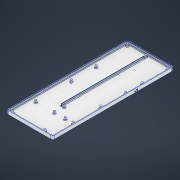
# Autodesk Inventor part: Base
Saved by Autodesk Inventor 2022 (Build 260153000, 153)
## iProperties
Created: 2021-09-21
Part Number: Base
Material: アルミニウム 6061
Document SubType Name: Modeling
Designer: shiok
Density: 2.7 g/cm^3
Appearance: アルミニウム - フラット
Author: shiok
Autodesk Inventor part; units mm, degrees
ref_plane "YZ Plane" through (0, 0, 0) normal (1, 0, 0) x (0, 1, 0)
ref_plane "XZ Plane" through (0, 0, 0) normal (0, 1, 0) x (-1, 0, 0)
ref_plane "XY Plane" through (0, 0, 0) normal (0, 0, 1) x (1, 0, 0)
ref_plane "作業平面5" through (0, 0, 0) normal (0, -1, 0) x (1, 0, 0)
sketch "スケッチ16" plane through (0, 0, 0) normal (0, -1, 0) x (1, 0, 0)
  line L0 (-65.58, -185.7375) -> (65.58, -185.7375)
  line L1 (71.12, -180.1975) -> (71.12, 180.1975)
  line L2 (65.58, 185.7375) -> (-65.58, 185.7375)
  line L3 (-71.12, 180.1975) -> (-71.12, -180.1975)
  arc A0 (-71.12, -180.1975) -> (-65.58, -185.7375) centre (-65.58, -180.1975) ccw
  arc A1 (65.58, -185.7375) -> (71.12, -180.1975) centre (65.58, -180.1975) ccw
  arc A2 (71.12, 180.1975) -> (65.58, 185.7375) centre (65.58, 180.1975) ccw
  arc A3 (-65.58, 185.7375) -> (-71.12, 180.1975) centre (-65.58, 180.1975) ccw
  line L4 (-65.58, -180.1975) -> (65.58, 180.1975)
  line L5 (-65.58, 180.1975) -> (65.58, -180.1975)
  point P0 (0, 0)
  point P1 (71.12, 185.7375)
  point P2 (71.12, -185.7375)
  point P3 (-71.12, 185.7375)
  point P4 (0, 0)
  point P5 (0, 0)
  dimension "d108" = 142.24
  dimension "d109" = 371.475
  dimension "d110" = 5.54
  constraints: 12 end point, 8 point on circle, 8 tangent, 6 point on line, 4 centre point, 3 equal radius, 3 midpoint, 2 parallel, 1 coincident, 1 horizontal, 1 perpendicular
  measures "d108" distance of point (-71.12, 185.738) point (71.12, 185.738)
  measures "d109" distance of point (71.12, 185.738) point (71.12, -185.738)
  measures "d110" radius of A0
extrude "押し出し12" add sketch "スケッチ16" against normal blind 2.54
sketch "スケッチ17" plane through (0, 2.54, 0) normal (0, 1, 0) x (1, 0, 0)
  line L0 (65.58, 183.1975) -> (-65.58, 183.1975)
  line L1 (-68.58, 180.1975) -> (-68.58, -180.1975)
  line L2 (-65.58, -183.1975) -> (65.58, -183.1975)
  line L3 (68.58, -180.1975) -> (68.58, 180.1975)
  arc A0 (68.58, 180.1975) -> (65.58, 183.1975) centre (65.58, 180.1975) ccw
  arc A1 (65.58, -183.1975) -> (68.58, -180.1975) centre (65.58, -180.1975) ccw
  arc A2 (-68.58, -180.1975) -> (-65.58, -183.1975) centre (-65.58, -180.1975) ccw
  arc A3 (-65.58, 183.1975) -> (-68.58, 180.1975) centre (-65.58, 180.1975) ccw
  line L4 (71.12, 180.1975) -> (71.12, -180.1975)
  arc A4 (65.58, -185.7375) -> (71.12, -180.1975) centre (65.58, -180.1975) ccw
  line L5 (65.58, -185.7375) -> (-65.58, -185.7375)
  arc A5 (-71.12, -180.1975) -> (-65.58, -185.7375) centre (-65.58, -180.1975) ccw
  line L6 (-71.12, -180.1975) -> (-71.12, 180.1975)
  arc A6 (-65.58, 185.7375) -> (-71.12, 180.1975) centre (-65.58, 180.1975) ccw
  line L7 (-65.58, 185.7375) -> (65.58, 185.7375)
  arc A7 (71.12, 180.1975) -> (65.58, 185.7375) centre (65.58, 180.1975) ccw
  line L8 (-65.58, 180.1975) -> (65.58, -180.1975) construction
  line L9 (-65.58, -180.1975) -> (65.58, 180.1975) construction
  circle A8 centre (62.23, 176.8475) radius 3
  circle A9 centre (63.5, 96.8375) radius 3
  circle A10 centre (63.5, 46.0375) radius 3
  circle A11 centre (62.23, -28.8925) radius 3
  circle A12 centre (62.23, -113.9825) radius 3
  circle A13 centre (38.1, -113.9825) radius 3
  circle A14 centre (38.1, -176.8475) radius 3
  circle A15 centre (-62.23, -176.8475) radius 3
  circle A16 centre (4.445, -113.9825) radius 3
  circle A17 centre (4.445, -83.5025) radius 3
  circle A18 centre (-52.705, -113.9825) radius 3
  circle A19 centre (-52.705, -4.7625) radius 3
  circle A20 centre (-52.705, 71.4375) radius 3
  circle A21 centre (-62.23, 176.8475) radius 3
  circle A22 centre (-5.08, 176.8475) radius 3
  point P0 (0, 0)
  point P1 (0, 0)
  point P2 (0, 0)
  point P3 (0, 0)
  point P4 (52.07, 166.6875)
  dimension "d113" = 3
  dimension "d114" = 2.54
  dimension "d115" = 366.395
  dimension "d116" = 137.16
  dimension "d117" = 16.51
  dimension "d118" = 16.51
  dimension "d119" = 10.16
  dimension "d120" = 10.16
  dimension "d121" = 1.27
  dimension "d122" = 1.27
  dimension "d123" = 80.01
  dimension "d124" = 50.8
  dimension "d125" = 74.93
  dimension "d126" = 85.09
  dimension "d127" = 6
  dimension "d128" = 6
  dimension "d129" = 6
  dimension "d130" = 6
  dimension "d131" = 6
  dimension "d132" = 24.13
  dimension "d133" = 62.865
  dimension "d134" = 100.33
  dimension "d135" = 62.865
  dimension "d136" = 9.525
  dimension "d137" = 6
  dimension "d138" = 6
  dimension "d139" = 57.15
  dimension "d140" = 76.2
  dimension "d141" = 6
  dimension "d142" = 6
  dimension "d143" = 109.22
  dimension "d144" = 6
  dimension "d145" = 6
  dimension "d146" = 6
  dimension "d147" = 6
  dimension "d148" = 6
  dimension "d149" = 6
  dimension "d150" = 30.48
  dimension "d151" = 33.655
  constraints: 23 centre point, 20 end point, 16 point on circle, 8 tangent, 7 vertical alignment, 5 horizontal alignment, 4 parallel, 3 equal radius, 3 midpoint, 2 perpendicular, 1 coincident, 1 horizontal, 7 other
  measures "d113" radius of A0
  measures "d114" distance between parallel lines of L3 L4
  measures "d115" distance between parallel lines of L2 L0
  measures "d116" distance between parallel lines of L1 L3
  measures "d117" distance from line of point (52.07, 166.688) L3
  measures "d118" distance from line of L0 point (52.07, 166.688)
  measures "d119" horizontal distance of A8.centre point (52.07, 166.688)
  measures "d120" horizontal distance of point (52.07, 166.688) A8.centre
  measures "d121" horizontal distance of A9.centre A8.centre
  measures "d122" horizontal distance of A11.centre A10.centre
  measures "d123" vertical distance of A9.centre A8.centre
  measures "d124" distance of A9.centre A10.centre
  measures "d125" vertical distance of A10.centre A11.centre
  measures "d126" distance of A12.centre A11.centre
  measures "d127" diameter of A8
  measures "d128" diameter of A9
  measures "d129" diameter of A10
  measures "d130" diameter of A11
  measures "d131" diameter of A12
  measures "d132" distance of A13.centre A12.centre
  measures "d133" distance of A14.centre A13.centre
  measures "d134" distance of A15.centre A14.centre
  measures "d135" vertical distance of A18.centre A15.centre
  measures "d136" horizontal distance of A18.centre A15.centre
  measures "d137" diameter of A21
  measures "d138" diameter of A22
  measures "d139" distance of A21.centre A22.centre
  measures "d140" distance of A19.centre A20.centre
  measures "d141" diameter of A20
  measures "d142" diameter of A19
  measures "d143" distance of A18.centre A19.centre
  measures "d144" diameter of A13
  measures "d145" diameter of A14
  measures "d146" diameter of A15
  measures "d147" diameter of A18
  measures "d148" diameter of A17
  measures "d149" diameter of A16
  measures "d150" distance of A17.centre A16.centre
  measures "d151" distance of A13.centre A16.centre
extrude "押し出し13" add sketch "スケッチ17" along normal blind 6.4 contours A8 | A9 | A10 | A11 | A12 | A13 | A14 | A15 | A16 | A17 | A18 | A19 | A20 | A21 | A22
sketch "スケッチ18" plane through (0, 2.54, 0) normal (0, 1, 0) x (1, 0, 0)
  line L0 (-65.58, -185.7375) -> (65.58, -185.7375)
  line L1 (71.12, -180.1975) -> (71.12, 180.1975)
  line L2 (65.58, 185.7375) -> (-65.58, 185.7375)
  line L3 (-71.12, 180.1975) -> (-71.12, -180.1975)
  arc A0 (-71.12, -180.1975) -> (-65.58, -185.7375) centre (-65.58, -180.1975) ccw
  arc A1 (65.58, -185.7375) -> (71.12, -180.1975) centre (65.58, -180.1975) ccw
  arc A2 (71.12, 180.1975) -> (65.58, 185.7375) centre (65.58, 180.1975) ccw
  arc A3 (-65.58, 185.7375) -> (-71.12, 180.1975) centre (-65.58, 180.1975) ccw
  line L4 (-65.58, -180.1975) -> (65.58, 180.1975)
  line L5 (-65.58, 180.1975) -> (65.58, -180.1975)
  line L6 (68.58, 180.1975) -> (68.58, -180.1975)
  arc A4 (65.58, -183.1975) -> (68.58, -180.1975) centre (65.58, -180.1975) ccw
  line L7 (65.58, -183.1975) -> (-65.58, -183.1975)
  arc A5 (-68.58, -180.1975) -> (-65.58, -183.1975) centre (-65.58, -180.1975) ccw
  line L8 (-68.58, -180.1975) -> (-68.58, 180.1975)
  arc A6 (-65.58, 183.1975) -> (-68.58, 180.1975) centre (-65.58, 180.1975) ccw
  line L9 (-65.58, 183.1975) -> (65.58, 183.1975)
  arc A7 (68.58, 180.1975) -> (65.58, 183.1975) centre (65.58, 180.1975) ccw
  point P0 (0, 0)
  point P1 (0, 0)
  point P2 (71.12, 185.7375)
  point P3 (71.12, -185.7375)
  point P4 (-71.12, 185.7375)
  point P5 (0, 0)
  point P6 (0, 0)
  dimension "d154" = 142.24
  dimension "d155" = 371.475
  dimension "d156" = 5.54
  dimension "d157" = 2.54
  constraints: 20 end point, 16 point on circle, 8 centre point, 8 tangent, 6 point on line, 4 parallel, 3 equal radius, 3 midpoint, 2 perpendicular, 1 coincident, 1 horizontal, 7 other
  measures "d154" distance of point (-71.12, 185.738) point (71.12, 185.738)
  measures "d155" distance of point (71.12, 185.738) point (71.12, -185.738)
  measures "d156" radius of A0
  measures "d157" distance between parallel lines of L1 L6
extrude "押し出し14" add sketch "スケッチ18" along normal blind 8
fillet "フィレット6" radius 1.5 23 edges at (67.7013, 2.54, -182.3188) (0, 2.54, -183.1975) (-67.7013, 2.54, -182.3188) (-68.58, 2.54, 0) (-67.7013, 2.54, 182.3188) (0, 2.54, 183.1975) (67.7013, 2.54, 182.3188) (68.58, 2.54, 0) (35.1, 2.54, 176.8475) (59.23, 2.54, 113.9825) (35.1, 2.54, 113.9825) (1.445, 2.54, 83.5025) (1.445, 2.54, 113.9825) (-65.23, 2.54, 176.8475) (-55.705, 2.54, 113.9825) (-55.705, 2.54, 4.7625) (59.23, 2.54, 28.8925) (60.5, 2.54, -46.0375) (60.5, 2.54, -96.8375) (59.23, 2.54, -176.8475) (-8.08, 2.54, -176.8475) (-65.23, 2.54, -176.8475) (-55.705, 2.54, -71.4375)
chamfer "面取り3" distance 0.5 angle 45 8 edges at (67.7013, 10.54, -182.3188) (68.58, 10.54, 0) (67.7013, 10.54, 182.3188) (0, 10.54, 183.1975) (-67.7013, 10.54, 182.3188) (-68.58, 10.54, 0) (-67.7013, 10.54, -182.3188) (0, 10.54, -183.1975)
sketch "スケッチ20" plane through (-5.08, 8.94, -176.8475) normal (0, 1, 0) x (1, 0, 0)
  line L0 (1.905, -7.62) -> (1.27, -7.62)
  line L1 (1.27, -7.62) -> (1.27, -260.35)
  line L2 (1.27, -260.35) -> (1.905, -260.35)
  line L3 (1.905, -260.35) -> (1.905, -7.62)
  line L4 (0.635, -7.62) -> (1.27, -7.62)
  line L5 (1.27, -260.35) -> (0.635, -260.35)
  line L6 (0.635, -260.35) -> (0.635, -7.62)
  point P0 (5.08, -176.8475)
  point P1 (0, 0)
  point P2 (0, 0)
  dimension "d164" = 0.635
  dimension "d165" = 252.73
  dimension "d166" = 7.62
  dimension "d167" = 1.27
  constraints: 14 end point, 2 parallel, 2 symmetric about line, 1 coincident, 1 horizontal, 1 perpendicular, 1 other
  measures "d164" distance of L2.end L1.end
  measures "d165" distance of L1.end L0.end
  measures "d166" distance from line of L0 point (0, 0)
  measures "d167" distance from line of point (0, 0) L1
extrude "押し出し15" add sketch "スケッチ20" against normal up to surface (6.4 mm away)
fillet "フィレット7" radius 2 4 edges at (-4.445, 2.54, -42.8625) (-3.175, 2.54, -42.8625) (-3.81, 2.54, -169.2275) (-3.81, 2.54, 83.5025)
sketch "スケッチ21" plane through (71.12, 0, 180.1975) normal (1, 0, 0) x (0, 0, -1)
  line L0 (247.392, 5.84) -> (255.892, 5.84)
  line L1 (255.892, 5.84) -> (255.892, 2.54)
  line L2 (255.892, 2.54) -> (247.392, 2.54)
  line L3 (247.392, 2.54) -> (247.392, 5.84)
  line L4 (365.935, 0) -> (365.935, 10.54) projected
  line L5 (360.395, 0) -> (0, 0) projected
  point P0 (180.1975, 0)
  dimension "d171" = 8.5
  dimension "d172" = 3.3
  dimension "d173" = 110.043
  dimension "d174" = 2.54
  constraints: 8 end point, 2 parallel, 1 horizontal, 1 perpendicular
  measures "d171" distance of L1.end L2.end
  measures "d172" distance of L0.end L1.end
  measures "d173" distance between parallel lines of L4 L1
  measures "d174" distance between parallel lines of L5 L2
extrude "押し出し16" cut sketch "スケッチ21" against normal blind 10
fillet "フィレット8" radius 0.5 4 edges at (69.1, 2.54, -67.1945) (69.1, 2.54, -75.6945) (69.85, 5.84, -67.1945) (69.85, 5.84, -75.6945)
chamfer "面取り4" distance 0.5 angle 45 8 edges at (71.12, 5.84, -71.4445) (71.12, 5.6936, -75.5481) (71.12, 4.19, -75.6945) (71.12, 2.6864, -75.5481) (71.12, 2.54, -71.4445) (71.12, 2.6864, -67.3409) (71.12, 4.19, -67.1945) (71.12, 5.6936, -67.3409)
fillet "フィレット9" radius 0.5 8 edges at (-2.5892, 3.1258, 84.0883) (-3.175, 6.74, 83.5025) (-5.0308, 3.1258, 84.0883) (-4.445, 6.74, 83.5025) (-2.5892, 3.1258, -169.8133) (-3.175, 6.74, -169.2275) (-5.0308, 3.1258, -169.8133) (-4.445, 6.74, -169.2275)
